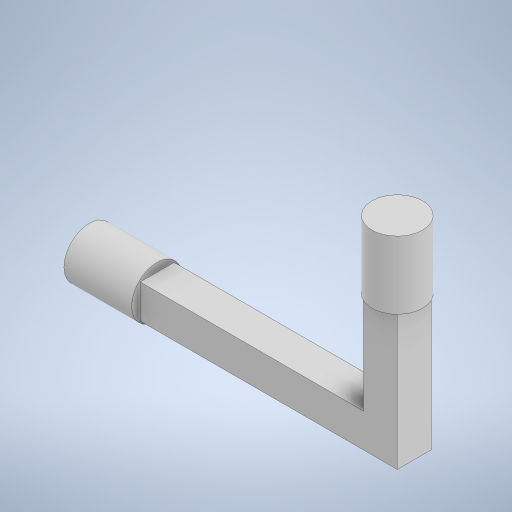
# Autodesk Inventor part: link_wr2wp_l
Saved by Autodesk Inventor 2024.3 (Build 283343000, 343)
## iProperties
Created: 2025-01-19
Part Number: link_wr2wp_l
Material: 一般
Document SubType Name: Modeling
Designer: yuu53
Density: 1 g/cm^3
Appearance: 既定
Author: yuu53
Autodesk Inventor part; units mm, degrees
ref_plane "YZ Plane" through (0, 0, 0) normal (1, 0, 0) x (0, 1, 0)
ref_plane "XZ Plane" through (0, 0, 0) normal (0, 1, 0) x (-1, 0, 0)
ref_plane "XY Plane" through (0, 0, 0) normal (0, 0, 1) x (1, 0, 0)
sketch "スケッチ1" plane through (0, 0, 0) normal (0, 0, 1) x (1, 0, 0)
  line L0 (-86, 5) -> (-86, -5)
  line L1 (-86, -5) -> (10, -5)
  line L2 (10, -5) -> (10, 55)
  line L3 (10, 55) -> (0, 55)
  line L4 (0, 55) -> (0, 5)
  line L5 (0, 5) -> (-86, 5)
  point P0 (0, 0)
  dimension "d0" = 10
  dimension "d1" = 10
  dimension "d2" = 60
  dimension "d3" = 10
  dimension "d4" = 96
  dimension "d5" = 5
  constraints: 12 end point, 5 perpendicular, 1 vertical
  measures "d0" distance of L0.start L0.end
  measures "d1" distance of L2.end L3.end
  measures "d2" distance of L1.end L2.end
  measures "d3" distance from line of L2 point (0, 0)
  measures "d4" distance of L0.end L1.end
  measures "d5" distance from line of L5 point (0, 0)
extrude "押し出し1" add sketch "スケッチ1" along normal blind 5 and the other way blind 5
sketch "スケッチ2" plane through (0, 55, 5) normal (0, 1, 0) x (1, 0, 0)
  circle A0 centre (5, 5) radius 7.5
  line L0 (0, 10) -> (10, 10) projected
  line L1 (0, 10) -> (0, 0) projected
  point P0 (0, 5)
  point P1 (0, 5)
  dimension "d10" = 5
  dimension "d11" = 5
  dimension "d12" = 15
  constraints: 1 centre point, 1 midpoint
  measures "d10" distance from line of A0.centre L0
  measures "d11" distance of point (0, 5) A0.centre
  measures "d12" diameter of A0
extrude "押し出し2" add sketch "スケッチ2" against normal blind 20
sketch "スケッチ3" plane through (-86, -5, 5) normal (-1, 0, 0) x (0, 0, 1)
  circle A0 centre (-5, 5) radius 7.5
  point P0 (-5, 5)
  dimension "d15" = 15
  constraints: 1 centre point, 1 coincident
  measures "d15" diameter of A0
extrude "押し出し3" add sketch "スケッチ3" against normal blind 20
